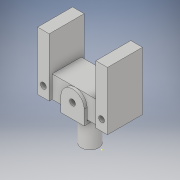
# Autodesk Inventor part: pinza
Saved by Autodesk Inventor 2019 (Build 230136000, 136)
## iProperties
Created: 2019-10-18
Part Number: pinza
Material: Genérico
Document SubType Name: Modeling
Designer: Josue
Density: 1 g/cm^3
Appearance: Valor por defecto
Author: Josue
Autodesk Inventor part; units mm, degrees
ref_plane "YZ Plane" through (0, 0, 0) normal (1, 0, 0) x (0, 1, 0)
sketch "Boceto1" plane through (0, 0, 0) normal (0, 1, 0) x (-1, 0, 0)
  circle A0 centre (0, 0) radius 15
  dimension "d0" = 30
  constraints: 1 centre point, 1 coincident
  measures "d0" diameter of A0
extrude "Extrusión1" add sketch "Boceto1" along normal blind 50
sketch "Boceto2" plane through (0, 50, 0) normal (0, 1, 0) x (1, 0, 0)
  line L0 (20, 30) -> (-20, 30)
  line L1 (-20, 30) -> (-20, -30)
  line L2 (-20, -30) -> (20, -30)
  line L3 (20, -30) -> (20, 30)
  line L4 (20, 30) -> (-20, -30) construction
  line L5 (-20, 30) -> (20, -30) construction
  point P0 (0, 0)
  dimension "d3" = 60
  dimension "d4" = 40
  constraints: 12 end point, 2 midpoint, 2 parallel, 1 horizontal, 1 perpendicular
  measures "d3" distance of L1.end L0.end
  measures "d4" distance of L0.start L0.end
extrude "Extrusión2" add sketch "Boceto2" along normal blind 5
sketch "Boceto3" plane through (-20, 50, 30) normal (0, 0, 1) x (1, 0, 0)
  line L0 (0, 5) -> (0, 25)
  line L1 (40, 5) -> (0, 5) projected
  line L2 (40, 5) -> (40, 25)
  arc A0 (40, 25) -> (0, 25) centre (20, 25) ccw
  circle A1 centre (20, 25) radius 5
  point P0 (20, -50)
  dimension "d7" = 20
  dimension "d8" = 20
  dimension "d9" = 10
  constraints: 4 end point, 2 centre point, 2 point on circle, 2 vertical, 1 coincident, 1 tangent
  measures "d7" distance of L0.start L0.end
  measures "d8" distance of L1.start L2.end
  measures "d9" diameter of A1
extrude "Extrusión3" add sketch "Boceto3" against normal blind 5
sketch "Boceto4" plane through (20, 50, -30) normal (0, 0, -1) x (-1, 0, 0)
  circle A0 centre (20, 25) radius 5 projected
  arc A1 (40, 25) -> (0, 25) centre (20, 25) ccw projected
  line L0 (40, 5) -> (40, 25) projected
  line L1 (0, 5) -> (40, 5) projected
  line L2 (0, 25) -> (0, 5) projected
  point P0 (20, -50)
extrude "Extrusión4" add sketch "Boceto4" against normal blind 5
sketch "Boceto5" plane through (20, 50, 30) normal (1, 0, 0) x (0, 0, -1)
  point P0 (30, -50)
ref_plane "Plano de trabajo1" through (0, 50, 30) normal (1, 0, 0) x (0, 0, -1)
ref_plane "Plano de trabajo2" through (-20, 50, 0) normal (0, 0, 1) x (1, 0, 0)
sketch "Boceto6" plane through (0, 50, 30) normal (1, 0, 0) x (0, 0, -1)
  line L0 (5, 25) -> (5, 45) projected
  line L1 (55, 7) -> (5, 7)
  line L2 (5, 7) -> (5, 45)
  line L3 (5, 45) -> (55, 45)
  line L4 (55, 45) -> (55, 7)
  line L5 (55, 7) -> (5, 45) construction
  line L6 (5, 7) -> (55, 45) construction
  point P0 (30, -50)
  point P1 (30, 26)
  constraints: 12 end point, 2 midpoint, 2 parallel, 1 horizontal, 1 perpendicular
extrude "Extrusión5" add sketch "Boceto6" along normal mid plane 120
sketch "Boceto7" plane through (20, 50, -30) normal (0, 0, -1) x (-1, 0, 0)
  circle A0 centre (20, 25) radius 5 projected
  point P0 (20, -50)
extrude "Extrusión6" cut sketch "Boceto7" against normal up to next
sketch "Boceto8" plane through (60, 50, 30) normal (1, 0, 0) x (0, 0, -1)
  line L0 (55, 7) -> (55, 5) projected
  line L1 (55, 7) -> (60, 7)
  line L2 (60, 7) -> (60, 107)
  line L3 (0, 7) -> (0, 107)
  line L4 (0, 107) -> (60, 107)
  line L5 (5, 25) -> (5, 7) projected
  line L6 (0, 7) -> (5, 7)
  line L7 (5, 7) -> (5, 45)
  line L8 (55, 45) -> (5, 45) projected
  line L9 (5, 45) -> (55, 45)
  line L10 (55, 45) -> (55, 7)
  point P0 (30, -50)
  dimension "d23" = 100
  constraints: 16 end point, 4 perpendicular, 1 horizontal, 1 vertical
  measures "d23" distance of L1.end L2.end
extrude "Extrusión7" add sketch "Boceto8" against normal blind 20
sketch "Boceto9" plane through (60, 57, -30) normal (0, 0, -1) x (-1, 0, 0)
  circle A0 centre (10, 18) radius 5
  point P0 (60, -57)
  dimension "d27" = 10
  constraints: 1 centre point
  measures "d27" diameter of A0
extrude "Extrusión8" cut sketch "Boceto9" against normal up to next
sketch "Boceto10" plane through (-60, 50, 30) normal (-1, 0, 0) x (0, 0, 1)
  line L0 (-60, 107) -> (-60, 7) projected
  line L1 (-5, 45) -> (-55, 45) projected
  line L2 (0, 107) -> (-60, 107) projected
  line L3 (-60, 7) -> (-55, 7) projected
  line L4 (-55, 45) -> (-55, 7) projected
  line L5 (-5, 45) -> (-55, 45) projected
  line L6 (-5, 7) -> (-5, 45) projected
  line L7 (-5, 7) -> (0, 7) projected
  line L8 (0, 7) -> (0, 107) projected
  line L9 (0, 107) -> (-60, 107) projected
  line L10 (-60, 107) -> (-60, 7) projected
  point P0 (-30, -50)
extrude "Extrusión9" add sketch "Boceto10" against normal blind 20
sketch "Boceto11" plane through (-60, 57, 30) normal (0, 0, 1) x (1, 0, 0)
  circle A0 centre (10, 18) radius 5
  point P0 (60, -57)
  dimension "d33" = 10
  constraints: 1 centre point
  measures "d33" diameter of A0
extrude "Extrusión10" cut sketch "Boceto11" against normal up to next
